# Autodesk Inventor part: LED-IR-THRUTSAL6100
Saved by Autodesk Inventor 2016 SP1 (Build 200210100, 210)
## iProperties
Created: 2015-11-19
Part Number: LED-IR-THRUTSAL6100
Material: Generic
Document SubType Name: Modeling
Designer: PhillipD
Density: 1 g/cm^3
Appearance: LED5MM, LED-IR-THRUTSAL6100
Author: PhillipD
Autodesk Inventor part; units mm, degrees
ref_plane "YZ Plane" through (0, 0, 0) normal (1, 0, 0) x (0, 1, 0)
ref_plane "XZ Plane" through (0, 0, 0) normal (0, 1, 0) x (-1, 0, 0)
ref_plane "XY Plane" through (0, 0, 0) normal (0, 0, 1) x (1, 0, 0)
sketch "LED5MM, LED-IR-THRUTSAL6100_13" plane through (0, 0, 0) normal (0, 0, 1) x (1, 0, 0)
  line L0 (-2.6162, 3.302) -> (2.6416, 3.302)
  line L1 (2.6416, 3.302) -> (2.6416, -2.6162)
  line L2 (2.6416, -2.6162) -> (-2.6162, -2.6162)
  line L3 (-2.6162, -2.6162) -> (-2.6162, 3.302)
  constraints: 8 end point
extrude "Extrusion1" add sketch "LED5MM, LED-IR-THRUTSAL6100_13" along normal blind 1
body "Solid1"
